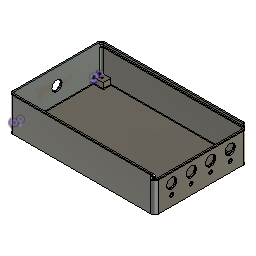
boite_alim_4x18650 (Autodesk Fusion 360 design; units mm, degrees)
Autodesk Fusion 360 part; units mm, degrees
sketch "Esquisse1" plane through (0, 0, 0) normal (0, 0, 1) x (1, 0, 0) in component "boite"
  line L0 (71, 47.5) -> (-71, 47.5)
  line L1 (-75, 43.5) -> (-75, -43.5)
  line L2 (-71, -47.5) -> (71, -47.5)
  line L3 (75, -43.5) -> (75, 43.5)
  line L4 (75, 47.5) -> (-75, -47.5) construction
  line L5 (-75, 47.5) -> (75, -47.5) construction
  arc A0 (-71, 47.5) -> (-75, 43.5) centre (-71, 43.5) ccw
  arc A1 (-75, -43.5) -> (-71, -47.5) centre (-71, -43.5) ccw
  arc A2 (75, 43.5) -> (71, 47.5) centre (71, 43.5) ccw
  arc A3 (71, -47.5) -> (75, -43.5) centre (71, -43.5) ccw
  dimension "d8" = 150
  dimension "d9" = 95
  dimension "d10" = 4
  constraint horizontal L0
  constraint perpendicular L0 L1
  constraint parallel L0 L2
  constraint parallel L1 L3
  constraint coincident L4 origin
  constraint coincident L5 origin
  constraint coincident L5.start L1
  constraint coincident L5.start L0
  constraint tangent L1 A0
  constraint tangent L0 A0
  constraint coincident L4.end L1
  constraint coincident L4.end L2
  constraint tangent L1 A1
  constraint tangent L2 A1
  constraint equal A0 A1
  constraint coincident L4.start L0
  constraint coincident L4.start L3
  constraint tangent L0 A2
  constraint tangent L3 A2
  constraint equal A0 A2
  constraint coincident L5.end L3
  constraint coincident L5.end L2
  constraint tangent L3 A3
  constraint tangent L2 A3
  constraint equal A0 A3
  measures "d8" distance of L4.end L5.end
  measures "d9" distance of L5.start L4.end
  measures "d10" radius of A0
extrude "Extrusion1" add sketch "Esquisse1" along normal blind 35.5 makes body 1 in component "boite"
sketch "Esquisse2" plane through (0, 0, 35.5) normal (0, 0, 1) x (-1, 0, 0) in component "boite"
  arc A0 (-71, 47.5) -> (-75, 43.5) centre (-71, 43.5) ccw
  line L0 (-75, 43.5) -> (-75, -43.5)
  arc A1 (-75, -43.5) -> (-71, -47.5) centre (-71, -43.5) ccw
  line L1 (-71, -47.5) -> (71, -47.5)
  arc A2 (71, -47.5) -> (75, -43.5) centre (71, -43.5) ccw
  line L2 (75, -43.5) -> (75, 43.5)
  arc A3 (75, 43.5) -> (71, 47.5) centre (71, 43.5) ccw
  line L3 (71, 47.5) -> (-71, 47.5)
  line L4 (-73, 43.5) -> (-73, -43.5)
  arc A4 (-73, -43.5) -> (-71, -45.5) centre (-71, -43.5) ccw
  line L5 (-71, -45.5) -> (71, -45.5)
  arc A5 (71, -45.5) -> (73, -43.5) centre (71, -43.5) ccw
  line L6 (73, -43.5) -> (73, 43.5)
  arc A6 (73, 43.5) -> (71, 45.5) centre (71, 43.5) ccw
  line L7 (71, 45.5) -> (-71, 45.5)
  arc A7 (-71, 45.5) -> (-73, 43.5) centre (-71, 43.5) ccw
extrude "Extrusion2" cut sketch "Esquisse2" against normal blind 33.5 contours L4 A4 L5 A5 L6 A6 L7 A7 bodies 1 in component "boite"
sketch "Esquisse3" plane through (75, 0, 0) normal (1, 0, 0) x (0, 1, 0) in component "boite"
  line L0 (-43.5, 0) -> (43.5, 0)
  line L1 (43.5, 0) -> (43.5, 35.5)
  line L2 (43.5, 35.5) -> (-43.5, 35.5)
  line L3 (-43.5, 35.5) -> (-43.5, 0)
  line L4 (-46.5, 33.5) -> (46.5, 33.5)
  line L5 (46.5, 33.5) -> (46.5, 31.2)
  line L6 (46.5, 31.2) -> (-46.5, 31.2)
  line L7 (-46.5, 31.2) -> (-46.5, 33.5)
  line L8 (-46.5, 33.5) -> (46.5, 31.2) construction
  line L9 (46.5, 33.5) -> (-46.5, 31.2) construction
  line L10 (-47.5, 0) -> (-47.5, 35.5)
  line L11 (-45.5, 33.5) -> (45.5, 33.5)
  line L12 (45.5, 33.5) -> (45.5, 35.5)
  line L13 (45.5, 35.5) -> (-45.5, 35.5)
  line L14 (-45.5, 35.5) -> (-45.5, 33.5)
  line L15 (-45.5, 33.5) -> (45.5, 35.5) construction
  line L16 (45.5, 33.5) -> (-45.5, 35.5) construction
  line L17 (-43.5, 35.5) -> (43.5, 35.5)
  line L18 (47.5, 0) -> (47.5, 35.5)
  point P0 (0, 32.35)
  point P1 (0, 34.5)
  dimension "d16" = 93
  dimension "d17" = 2.3
  dimension "d18" = 2
  dimension "d68" = 47.5
  dimension "d136" = 2
  dimension "d137" = 2
  dimension "d138" = 2
  constraint horizontal L4
  constraint perpendicular L4 L5
  constraint parallel L4 L6
  constraint parallel L5 L7
  constraint coincident L8 P0
  constraint coincident L9 P0
  constraint horizontal L11
  constraint perpendicular L11 L12
  constraint parallel L11 L13
  constraint parallel L12 L14
  constraint coincident L15 P1
  constraint coincident L16 P1
  constraint coincident L13 L2.end
  measures "d16" distance of L4.start L4.end
  measures "d17" distance of L4.start L6.end
  measures "d18" distance of L2 L4
  measures "d68" distance of P0 L10
  measures "d136" distance of L10 L14
  measures "d137" distance of L12 L18
  measures "d138" distance of L11 L13
extrude "Extrusion3" cut sketch "Esquisse3" against normal blind 148 contours L3 L4 L6 L7 L11 | L1 L3 L4 L6 L11 | L1 L4 L5 L6 L11 | L3 L4 L11 L13 L14 | L1 L2 L3 L4 L11 L13 L17 | L1 L4 L11 L12 L13 bodies 1 in component "boite"
fillet "Congé15" radius 2 2 edges at (-73, -45.5, 34.5) (-73, 45.5, 34.5) on bodies 1 in component "boite"
fillet "Congé16" radius 1.7 2 edges at (-73, -46.5, 32.35) (-73, 46.5, 32.35) on bodies 1 in component "boite"
sketch "Esquisse1 (2)" plane through (75, 0, 0) normal (1, 0, 0) x (0, 1, 0) in component "couvercle"
  line L0 (43.5, 31.2) -> (-43.5, 31.2)
  line L1 (-43.5, 31.2) -> (-43.5, 0)
  line L2 (-43.5, 0) -> (43.5, 0)
  line L3 (43.5, 0) -> (43.5, 31.2)
  line L4 (-46.2, 33.2) -> (46.2, 33.2)
  line L5 (46.2, 33.2) -> (46.2, 31.5)
  line L6 (46.2, 31.5) -> (-46.2, 31.5)
  line L7 (-46.2, 31.5) -> (-46.2, 33.2)
  line L8 (-46.2, 33.2) -> (46.2, 31.5) construction
  line L9 (46.2, 33.2) -> (-46.2, 31.5) construction
  line L10 (-46.5, 31.2) -> (-46.5, 33.5)
  line L11 (46.5, 33.5) -> (46.5, 31.2)
  line L12 (-45.5, 33.5) -> (-46.5, 33.5)
  line L13 (-46.5, 31.2) -> (-43.5, 31.2)
  line L14 (-30.7, 35.5) -> (30.7, 35.5)
  line L15 (30.7, 35.5) -> (30.7, 32.0889)
  line L16 (30.7, 32.0889) -> (-30.7, 32.0889)
  line L17 (-30.7, 32.0889) -> (-30.7, 35.5)
  line L18 (-30.7, 35.5) -> (30.7, 32.0889) construction
  line L19 (30.7, 35.5) -> (-30.7, 32.0889) construction
  line L20 (-31, 48) -> (-31, 50)
  line L21 (31, 48) -> (31, 50)
  line L22 (-43.5, 35.5) -> (43.5, 35.5)
  point P0 (0, 32.35)
  point P1 (0, 33.7944)
  dimension "d109" = 0.3
  dimension "d110" = 0.3
  dimension "d112" = 0.3
  dimension "d114" = 0.3
  dimension "d115" = 0.3
  dimension "d116" = 0.3
  constraint horizontal L4
  constraint perpendicular L4 L5
  constraint parallel L4 L6
  constraint parallel L5 L7
  constraint coincident L8 P0
  constraint coincident L9 P0
  constraint horizontal L14
  constraint perpendicular L14 L15
  constraint parallel L14 L16
  constraint parallel L15 L17
  constraint coincident L18 P1
  constraint coincident L19 P1
  constraint coincident L14.start L22
  measures "d109" distance of L7 L10
  measures "d110" distance of L5 L11
  measures "d112" distance of L4 L12
  measures "d114" distance of L6 L13
  measures "d115" distance of L17 L20
  measures "d116" distance of L15 L21
extrude "Extrusion1'" add sketch "Esquisse1 (2)" against normal up to surface (148 mm away) separate body contours L4 L5 L6 L7 L15 L16 L17 | L4 L15 L16 L17 makes body 2 in component "couvercle"
fillet "Congé1" radius 1.7 2 edges at (-73, -46.2, 32.35) (-73, 46.2, 32.35) on bodies 2 in component "couvercle"
sketch "Esquisse5" plane through (0, 0, 33.2) normal (0, 0, 1) x (-1, 0, 0) in component "couvercle"
  arc A0 (71.3, -46.2) -> (73, -44.5) centre (71.3, -44.5) ccw
  line L0 (73, -44.5) -> (73, 44.5)
  arc A1 (73, 44.5) -> (71.3, 46.2) centre (71.3, 44.5) ccw
  line L1 (71.3, 46.2) -> (-75, 46.2)
  line L2 (-75, 46.2) -> (-75, -46.2)
  line L3 (-75, -46.2) -> (71.3, -46.2)
  arc A2 (-71, 47.5) -> (-74.4641, 45.5) centre (-71, 43.5) ccw
  line L4 (-75, 46.2) -> (71.3, 46.2)
  line L5 (-75, 46.2) -> (-75, -46.2)
  line L6 (-75, -46.2) -> (71.3, -46.2)
  arc A3 (-74.4641, -45.5) -> (-71, -47.5) centre (-71, -43.5) ccw
  arc A4 (-75, -43.5) -> (-71, -47.5) centre (-71, -43.5) ccw
  arc A5 (-71, 47.5) -> (-75, 43.5) centre (-71, 43.5) ccw
sketch "Esquisse9" plane through (0, 0, 33.2) normal (0, 0, 1) x (-1, 0, 0)
  arc A0 (71.3, -46.2) -> (73, -44.5) centre (71.3, -44.5) ccw
  line L0 (73, -44.5) -> (73, 44.5)
  arc A1 (73, 44.5) -> (71.3, 46.2) centre (71.3, 44.5) ccw
  line L1 (71.3, 46.2) -> (-75, 46.2)
  line L2 (-75, 46.2) -> (-75, -46.2)
  line L3 (-75, -46.2) -> (71.3, -46.2)
  arc A2 (-75, -43.5) -> (-73.6458, -46.5) centre (-71, -43.5) ccw
  arc A3 (-73.6458, 46.5) -> (-75, 43.5) centre (-71, 43.5) ccw
extrude "Extrusion6" cut sketch "Esquisse9" against normal blind 2 contours L2 L3 A2 | L1 L2 A3 bodies 2 in component "couvercle"
sketch "Esquisse10" plane through (0, 0, 33.2) normal (0, 0, 1) x (-1, 0, 0)
  arc A0 (-75, -43.5) -> (-73.9513, -46.2) centre (-71, -43.5) ccw
  line L0 (-73.9513, -46.2) -> (71.3, -46.2)
  arc A1 (71.3, -46.2) -> (73, -44.5) centre (71.3, -44.5) ccw
  line L1 (73, -44.5) -> (73, 44.5)
  arc A2 (73, 44.5) -> (71.3, 46.2) centre (71.3, 44.5) ccw
  line L2 (71.3, 46.2) -> (-73.9513, 46.2)
  arc A3 (-73.9513, 46.2) -> (-75, 43.5) centre (-71, 43.5) ccw
  line L3 (-75, 43.5) -> (-75, -43.5)
  line L4 (-73, -45.2) -> (-75, -45.2)
  line L5 (-75, -45.2) -> (-75, 45.2)
  line L6 (-75, 45.2) -> (-73, 45.2)
  line L7 (-73, 45.2) -> (-73, -45.2)
  line L8 (-73, -45.2) -> (-75, 45.2) construction
  line L9 (-75, -45.2) -> (-73, 45.2) construction
  line L10 (-75, 43.5) -> (-75, -43.5)
  line L11 (71, -45.5) -> (-74.4641, -45.5)
  line L12 (-74.4641, 45.5) -> (71, 45.5)
  arc A4 (-75, -43.5) -> (-73.9513, -46.2) centre (-71, -43.5) ccw
  arc A5 (-73.9513, 46.2) -> (-75, 43.5) centre (-71, 43.5) ccw
  point P0 (-74, 0)
  dimension "d145" = 2
  dimension "d146" = 0.3
  dimension "d147" = 0.3
  constraint horizontal L4
  constraint perpendicular L4 L5
  constraint parallel L4 L6
  constraint parallel L5 L7
  constraint coincident L8 P0
  constraint coincident L9 P0
  constraint coincident A0.start L5
  measures "d145" distance of L5 L7
  measures "d146" distance of L4 L11
  measures "d147" distance of L6 L12
extrude "Extrusion7" add sketch "Esquisse10" along normal blind 2.3 contours A0 A3 L3 L4 L5 L6 L7 L10 A4 A5 bodies 2 in component "couvercle"
move_body "Déplacer2" bodies 2 to x (1, 0, 0) y (0, 1, 0) z (0, 0, 1) at (30, 0, 0) in component "couvercle"
sketch "Esquisse14" plane through (0, 0, 2) normal (0, 0, 1) x (-1, 0, 0)
  arc A0 (-71, 45.5) -> (-73, 43.5) centre (-71, 43.5) ccw
  line L0 (-73, 43.5) -> (-73, -43.5)
  arc A1 (-73, -43.5) -> (-71, -45.5) centre (-71, -43.5) ccw
  line L1 (-71, -45.5) -> (71, -45.5)
  arc A2 (71, -45.5) -> (73, -43.5) centre (71, -43.5) ccw
  line L2 (73, -43.5) -> (73, 43.5)
  arc A3 (73, 43.5) -> (71, 45.5) centre (71, 43.5) ccw
  line L3 (71, 45.5) -> (-71, 45.5)
  line L4 (-73, 45.5) -> (-63, 45.5)
  line L5 (-63, 45.5) -> (-63, 37.5)
  line L6 (-63, 37.5) -> (-73, 37.5)
  line L7 (-73, 37.5) -> (-73, 45.5)
  line L8 (-73.003, -45.5023) -> (-63.003, -45.5023)
  line L9 (-63.003, -45.5023) -> (-63.003, -37.5023)
  line L10 (-63.003, -37.5023) -> (-73.003, -37.5023)
  line L11 (-73.003, -37.5023) -> (-73.003, -45.5023)
  line L12 (73, 45.5) -> (63, 45.5)
  line L13 (63, 45.5) -> (63, 37.5)
  line L14 (63, 37.5) -> (73, 37.5)
  line L15 (73, 37.5) -> (73, 45.5)
  line L16 (73, -45.5) -> (63, -45.5)
  line L17 (63, -45.5) -> (63, -37.5)
  line L18 (63, -37.5) -> (73, -37.5)
  line L19 (73, -37.5) -> (73, -45.5)
  circle A4 centre (68, -41.5) radius 0.75
  circle A5 centre (68, 41.5) radius 0.75
  circle A6 centre (-68, 41.5) radius 0.75
  circle A7 centre (-68.003, -41.5023) radius 0.75
  dimension "d170" = 10
  dimension "d171" = 8
  dimension "d172" = 10
  dimension "d173" = 8
  dimension "d174" = 10
  dimension "d175" = 8
  dimension "d176" = 10
  dimension "d177" = 8
  dimension "d178" = 1.5
  dimension "d179" = 5
  dimension "d180" = 4
  dimension "d181" = 1.5
  dimension "d182" = 5
  dimension "d183" = 4
  dimension "d184" = 1.5
  dimension "d185" = 4
  dimension "d186" = 5
  dimension "d187" = 1.5
  dimension "d188" = 4
  dimension "d189" = 5
  constraint horizontal L4
  constraint vertical L5
  constraint horizontal L6
  constraint vertical L7
  constraint horizontal L8
  constraint vertical L9
  constraint horizontal L10
  constraint vertical L11
  constraint horizontal L12
  constraint vertical L13
  constraint horizontal L14
  constraint vertical L15
  constraint horizontal L16
  constraint vertical L17
  constraint horizontal L18
  constraint vertical L19
  measures "d170" distance of L4.start L4.end
  measures "d171" distance of L4.start L6.end
  measures "d172" distance of L8.start L8.end
  measures "d173" distance of L8.start L10.end
  measures "d174" distance of L12.start L12.end
  measures "d175" distance of L12.start L14.end
  measures "d176" distance of L16.start L16.end
  measures "d177" distance of L16.start L18.end
  measures "d178" diameter of A4
  measures "d179" distance of L19 A4.centre
  measures "d180" distance of L18 A4.centre
  measures "d181" diameter of A5
  measures "d182" distance of L13 A5.centre
  measures "d183" distance of L12 A5.centre
  measures "d184" diameter of A6
  measures "d185" distance of L4 A6.centre
  measures "d186" distance of L7 A6.centre
  measures "d187" diameter of A7
  measures "d188" distance of L8 A7.centre
  measures "d189" distance of L11 A7.centre
extrude "Extrusion8" add sketch "Esquisse14" along normal blind 5.8 contours A0 L0 L3 L4 L5 L6 L7 | L2 A3 L3 L12 L13 L14 L15 | L0 A1 L1 L9 L10 | L1 A2 L2 L16 L17 L18 L19 bodies 1 in component "boite"
sketch "Esquisse11" plane through (-73, 0, 0) normal (1, 0, 0) x (0, 1, 0)
  line L0 (44.8, 31.2) -> (44.8, 33.5)
  line L1 (44.8, 33.5) -> (43.5, 33.5)
  line L2 (43.5, 33.5) -> (43.5, 35.5)
  line L3 (43.5, 35.5) -> (-43.5, 35.5)
  line L4 (-43.5, 35.5) -> (-43.5, 33.5)
  line L5 (-43.5, 33.5) -> (-44.8, 33.5)
  line L6 (-44.8, 33.5) -> (-44.8, 31.2)
  line L7 (-44.8, 31.2) -> (-43.5, 31.2)
  line L8 (-43.5, 31.2) -> (-43.5, 7.8)
  line L9 (-37.5, 2) -> (37.5, 2)
  line L10 (43.5, 7.8) -> (43.5, 31.2)
  line L11 (43.5, 31.2) -> (44.8, 31.2)
  line L12 (-37.5, 7.8) -> (-37.5, 2)
  line L13 (37.5, 2) -> (37.5, 7.8)
  line L14 (37.5, 7.8) -> (43.5, 7.8)
  line L15 (-43.5, 7.8) -> (-37.5, 7.8)
sketch "Esquisse12" plane through (-75, 0, 0) normal (-1, 0, 0) x (0, -1, 0)
  line L0 (-43.5, 0) -> (43.5, 0)
  line L1 (43.5, 0) -> (43.5, 35.5)
  line L2 (43.5, 35.5) -> (-43.5, 35.5)
  line L3 (-43.5, 35.5) -> (-43.5, 0)
  circle A0 centre (0, 19) radius 4.75
  dimension "d150" = 9.5
  measures "d150" diameter of A0
extrude "Extrusion6'" cut sketch "Esquisse12" against normal blind 2 contours A0 bodies 1 in component "boite"
sketch "Esquisse13" plane through (75, 0, 0) normal (1, 0, 0) x (0, 1, 0)
  line L0 (43.5, 31.2) -> (-43.5, 31.2)
  line L1 (-43.5, 31.2) -> (-43.5, 0)
  line L2 (-43.5, 0) -> (43.5, 0)
  line L3 (43.5, 0) -> (43.5, 31.2)
  line L4 (-57.3208, 10.8) -> (73.3392, 10.8)
  circle A0 centre (-10, 10.8) radius 1.5
  circle A1 centre (-30, 10.8) radius 1.5
  circle A2 centre (10, 10.8) radius 1.5
  circle A3 centre (30, 10.8) radius 1.5
  line L5 (0, 2.5) -> (0, 20)
  line L6 (-55, 21.2) -> (55, 21.2)
  circle A4 centre (-30.0375, 21.2) radius 4.75
  circle A5 centre (-9.8747, 21.2) radius 4.75
  circle A6 centre (9.9915, 21.2) radius 4.75
  circle A7 centre (29.9882, 21.2) radius 4.75
  dimension "d154" = 10.8
  dimension "d155" = 3
  dimension "d156" = 3
  dimension "d157" = 3
  dimension "d158" = 3
  dimension "d159" = 10
  dimension "d160" = 20
  dimension "d161" = 20
  dimension "d162" = 20
  dimension "d163" = 10
  dimension "d164" = 9.5
  dimension "d165" = 9.5
  dimension "d166" = 9.5
  dimension "d167" = 9.5
  constraint perpendicular L3 L4
  constraint coincident L4 A0.centre
  constraint coincident L4 A1.centre
  constraint coincident L4 A2.centre
  constraint coincident L4 A3.centre
  constraint horizontal L6
  constraint coincident L6 A4.centre
  constraint coincident L6 A5.centre
  constraint coincident L6 A6.centre
  constraint coincident L6 A7.centre
  measures "d154" distance of L2 L4
  measures "d155" diameter of A0
  measures "d156" diameter of A1
  measures "d157" diameter of A2
  measures "d158" diameter of A3
  measures "d159" distance of A0.centre L5
  measures "d160" distance of A0.centre A1.centre
  measures "d161" distance of A0.centre A2.centre
  measures "d162" distance of A2.centre A3.centre
  measures "d163" distance of L0 L6
  measures "d164" diameter of A4
  measures "d165" diameter of A5
  measures "d166" diameter of A6
  measures "d167" diameter of A7
extrude "Extrusion7'" cut sketch "Esquisse13" against normal blind 2 contours L6 A7 | L6 A7 | L6 A4 | L6 A4 | L4 A3 | L4 A3 | L4 A1 | L4 A1 | L6 A6 | L6 A6 | L6 A5 | L6 A5 | L4 A2 | L4 A2 | L4 A0 | L4 A0 bodies 1 in component "boite"
fillet "Congé17" radius 0.5 30 edges at (75, -34.466, 22.9177) (75, -14.3033, 22.9177) (75, 5.563, 22.9177) (75, 25.5597, 22.9177) (-73, 4.4286, 17.2823) (75, 28.6015, 11.3424) (75, 8.6015, 11.3424) (75, -11.3985, 11.3424) (75, -31.3985, 11.3424) (73, 8.6015, 10.2576) (73, 28.6015, 10.2576) (73, 25.5597, 19.4823) (73, 5.563, 19.4823) (73, -14.3033, 19.4823) (73, -11.3985, 10.2576) (73, -31.3985, 10.2576) (73, -34.466, 19.4823) (-75, 4.4286, 20.7177) (-68, 37.5, 2) (-63, 41.5, 2) (68.0015, 37.5023, 2) (63.003, 41.5012, 2) (63, -41.5, 2) (68, -37.5, 2) (-68, -37.5, 2) (-63, -41.5, 2) (0, -45.5, 2) (-73, 0, 2) (73, 0.0012, 2) (0.0015, 45.5, 2) 8 faces at (-75, -30.5833, 18.1667) (-71.1903, -47.4955, 23.6667) (-23.6667, -47.5, 11.8333) (73.0547, -46.9319, 23.6667) (75, 3.296, 3.1014) (73.0547, 46.9319, 23.6667) (23.6667, 47.5, 11.8333) (-73, 46.9641, 23.6667) on bodies 1 in component "boite"
component "boite" placed x (1, 0, 0) y (0, 1, 0) z (0, 0, 1) at (0, 0, 0)
component "couvercle" placed x (1, 0, 0) y (0, 1, 0) z (0, 0, 1) at (0, 0, 0)
equation "longueur = 150 mm"
equation "largeur = 95 mm"
equation "hauteur = 35.5 mm"
equation "epaisseur = 2 mm"
equation "rayonext = 4 mm"
equation "rayonint = rayonext - epaisseur"
equation "jeu = 0.3 mm"
equation "d8 = longueur"
equation "d9 = largeur"
equation "d10 = rayonext"
equation "d11 = hauteur"
equation "d13 = -epaisseur"
equation "d14 = -hauteur + epaisseur"
equation "d16 = largeur - epaisseur"
equation "d17 = jeu + epaisseur"
equation "d18 = epaisseur"
equation "d21 = -longueur + epaisseur"
equation "d68 = largeur / 2"
equation "d109 = jeu"
equation "d110 = jeu"
equation "d112 = jeu"
equation "d114 = jeu"
equation "d115 = jeu"
equation "d116 = jeu"
equation "d120 = rayonint - jeu"
equation "d136 = epaisseur"
equation "d137 = epaisseur"
equation "d138 = d18"
equation "d140 = rayonint"
equation "d142 = rayonint - jeu"
equation "d143 = -epaisseur"
equation "d146 = jeu"
equation "d147 = jeu"
equation "d148 = epaisseur + jeu"
equation "d151 = -epaisseur"
equation "d154 = d190 + 5 mm"
equation "d168 = -epaisseur"
equation "d190 = 5.8 mm"
